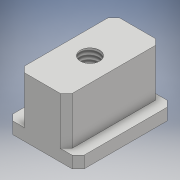
# Autodesk Inventor part: Peça1
Saved by Autodesk Inventor 2018 (Build 220112000, 112)
## iProperties
Created: 2018-08-28
Part Number: Peça1
Material: Genérico
Document SubType Name: Modeling
Designer: Georgines
Density: 1 g/cm^3
Appearance: Padrão
Author: Georgines
Autodesk Inventor part; units mm, degrees
ref_plane "YZ Plane" through (0, 0, 0) normal (1, 0, 0) x (0, 1, 0)
ref_plane "XZ Plane" through (0, 0, 0) normal (0, 1, 0) x (-1, 0, 0)
ref_plane "XY Plane" through (0, 0, 0) normal (0, 0, 1) x (1, 0, 0)
sketch "Esboço1" plane through (0, 0, 0) normal (0, 0, 1) x (1, 0, 0)
  line L0 (-6, 8) -> (6, 8)
  line L1 (6, 8) -> (6, -8)
  line L2 (6, -8) -> (-6, -8)
  line L3 (-6, -8) -> (-6, 8)
  line L4 (-6, 8) -> (6, -8) construction
  line L5 (6, 8) -> (-6, -8) construction
  point P0 (0, 0)
  dimension "d0" = 12
  dimension "d1" = 16
  constraints: 12 end point, 2 midpoint, 2 parallel, 1 horizontal, 1 perpendicular
  measures "d0" distance of L1.end L2.end
  measures "d1" distance of L0.end L1.end
extrude "Extrusão1" add sketch "Esboço1" along normal blind 10
sketch "Esboço3" plane through (0, 0, 10) normal (0, 0, 1) x (1, 0, 0)
  line L0 (6, -8) -> (-6, -8)
  line L1 (-6, -8) -> (-6, 8)
  line L2 (-6, 8) -> (6, 8)
  line L3 (6, 8) -> (6, -8)
  line L4 (6, -8) -> (-6, 8) construction
  line L5 (-6, -8) -> (6, 8) construction
  line L6 (4, -8) -> (-4, -8)
  line L7 (-4, -8) -> (-4, 8)
  line L8 (-4, 8) -> (4, 8)
  line L9 (4, 8) -> (4, -8)
  line L10 (4, -8) -> (-4, 8) construction
  line L11 (-4, -8) -> (4, 8) construction
  point P0 (0, 0)
  dimension "d4" = 12
  dimension "d5" = 16
  dimension "d6" = 8
  constraints: 24 end point, 4 midpoint, 4 parallel, 2 horizontal, 2 perpendicular, 1 point on line
  measures "d4" distance of L1.end L2.end
  measures "d5" distance of L0.end L1.end
  measures "d6" distance of L7.end L8.end
extrude "Extrusão2" cut sketch "Esboço3" against normal blind 8 contours L0 L9 L2 L3 | L0 L1 L2 L7
chamfer "Chanfro1" distance 1 angle 45 8 edges at (6, -8, 1) (-6, -8, 1) (6, 8, 1) (-6, 8, 1) (-4, -8, 6) (-4, 8, 6) (4, 8, 6) (4, -8, 6)
sketch "Esboço4" plane through (0, 0, 10) normal (0, 0, 1) x (1, 0, 0)
  circle A0 centre (0, 0) radius 1.5 construction
  dimension "d12" = 3
  constraints: 1 centre point, 1 coincident
  measures "d12" diameter of A0
hole "Furo1" at (0, 0, 10) direction (0, 0, -1) diameter 3.242 end through all thread size "M4x0.7" class "6H" standard "ANSI Metric M Profile"
